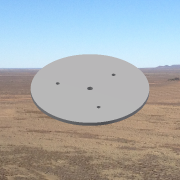
# Autodesk Inventor part: bpPlate
Saved by Autodesk Inventor 2014 SP1 (Build 180222100, 222)
## iProperties
Created: 2014-09-16
Part Number: bpPlate
Material: Steel
Document SubType Name: Modeling
Designer: Dave
Mass: 2424.78 g
Surface Area: 709.39 cm^2
Volume: 308.889 cm^3
Density: 7.85 g/cm^3
Appearance: Steel
Author: Dave
Autodesk Inventor part; units mm, degrees
ref_plane "YZ Plane" through (0, 0, 0) normal (1, 0, 0) x (0, 1, 0)
ref_plane "XZ Plane" through (0, 0, 0) normal (0, 1, 0) x (-1, 0, 0)
ref_plane "XY Plane" through (0, 0, 0) normal (0, 0, 1) x (1, 0, 0)
sketch "Sketch1" plane through (0, 0, 0) normal (0, 1, 0) x (-1, 0, 0)
  circle A0 centre (0, 0) radius 101.6
  dimension "d0" = 203.2
  constraints: 1 centre point, 1 coincident
  measures "d0" diameter of A0
extrude "Extrusion1" add sketch "Sketch1" along normal blind 6.35
sketch "Sketch2" plane through (0, 6.35, 0) normal (0, 1, 0) x (1, 0, 0)
  circle A0 centre (0, 0) radius 101.6 projected
  circle A1 centre (0, 0) radius 6.35
  dimension "d3" = 12.7
  constraints: 1 centre point, 1 coincident
  measures "d3" diameter of A1
hole "Hole1" at (0, 6.35, 0) direction (0, -1, 0) diameter 10.0838 end through all clearance for "Flat Head Machine Screw (82)" size "3/8" standard "Ansi Unified Screw Threads"
sketch "Sketch4" plane through (0, 6.35, 0) normal (0, 1, 0) x (1, 0, 0)
  circle A0 centre (0, 0) radius 5.0419 projected
  circle A1 centre (0, 57.15) radius 3.175
  circle A2 centre (-49.4934, -28.575) radius 3.175
  circle A3 centre (49.4934, -28.575) radius 3.175
  dimension "d24" = 6.35
  dimension "d25" = 57.15
  dimension "d28" = 360
  constraints: 3 centre point, 7 other
  measures "d24" diameter of A1
  measures "d25" distance of A0.centre A1.centre
hole "Hole3" at (0, 6.35, -57.15) at (49.4934, 6.35, 28.575) at (-49.4934, 6.35, 28.575) direction (0, -1, 0) diameter 6.7564 end through all clearance for "Flat Head Machine Screw (82)" size "1/4" standard "Ansi Unified Screw Threads"
body "Solid1"
